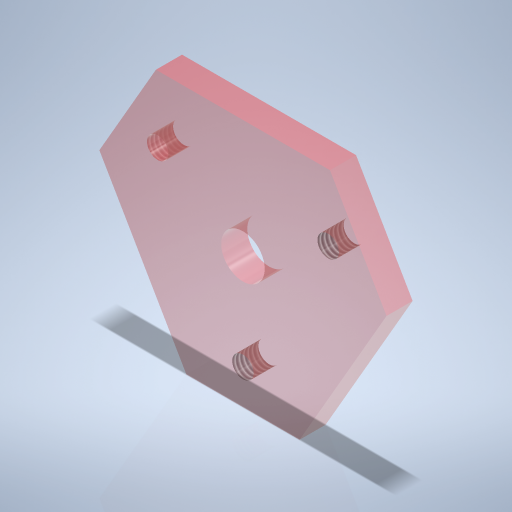
# Autodesk Inventor part: Plate
Saved by Autodesk Inventor 2024 (Build 280153000, 153)
## iProperties
Created: 2024-06-06
Part Number: Plate
Material: Aluminium 6061
Document SubType Name: Modeling
Designer: ffogue
Density: 2.7 g/cm^3
Appearance: Dunkelrot
Author: ffogue
Autodesk Inventor part; units mm, degrees
ref_plane "YZ Plane" through (0, 0, 0) normal (1, 0, 0) x (0, 1, 0)
ref_plane "XZ Plane" through (0, 0, 0) normal (0, 1, 0) x (-1, 0, 0)
ref_plane "XY Plane" through (0, 0, 0) normal (0, 0, 1) x (1, 0, 0)
sketch "Skizze1" plane through (0, 0, 0) normal (0, 1, 0) x (-1, 0, 0)
  line L0 (0, 0) -> (46, 79.6743)
  line L1 (46, 79.6743) -> (-46, 79.6743)
  line L2 (-46, 79.6743) -> (0, 0)
  line L3 (0, 0) -> (0, 79.6743) construction
  line L4 (-46, 79.6743) -> (23, 39.8372) construction
  line L5 (46, 79.6743) -> (-23, 39.8372) construction
  dimension "d0" = 92
  constraints: 12 end point, 3 midpoint, 1 equal length, 1 horizontal, 1 symmetric about line, 1 vertical
  measures "d0" distance of L1.end L0.start
extrude "Extrusion1" add sketch "Skizze1" along normal mid plane 6
sketch "Skizze2" plane through (0, -3, 0) normal (0, -1, 0) x (1, 0, 0)
  line L0 (46, 79.6743) -> (-46, 79.6743) projected
  line L1 (-46, 79.6743) -> (0, 0) projected
  line L2 (0, 0) -> (46, 79.6743) projected
  line L3 (0, 0) -> (0, 0) construction
  line L4 (0, 0) -> (0, 79.6743) construction
  line L5 (-46, 79.6743) -> (0, 0) projected
  line L6 (46, 79.6743) -> (-46, 79.6743) projected
  line L7 (-23, 39.8372) -> (46, 79.6743) construction
  line L8 (23, 39.8372) -> (-46, 79.6743) construction
  line L9 (-33, 57.1577) -> (-20, 79.6743)
  point P0 (-33, 57.1577)
  point P1 (-20, 79.6743)
  point P2 (-26.5, 68.416)
  dimension "d31" = 26
  constraints: 10 end point, 4 midpoint, 3 point on line, 1 perpendicular, 1 vertical
  measures "d31" distance of L9.start L9.end
extrude "Extrusion6" cut sketch "Skizze2" against normal blind 10 contours L9 L1 L0
mirror "Spiegeln1" about plane through (0, 0, 0) normal (1, 0, 0) of "Extrusion6"
sketch "Skizze7" plane through (0, -3, 0) normal (0, -1, 0) x (1, 0, 0)
  line L0 (0, 0) -> (-33, 57.1577) projected
  line L1 (-13, 22.5167) -> (13, 22.5167)
  line L2 (33, 57.1577) -> (0, 0) projected
  dimension "d38" = 26
  constraints: 2 end point, 2 point on line, 1 horizontal
  measures "d38" distance of L1.start L1.end
extrude "Extrusion7" cut sketch "Skizze7" against normal blind 10
sketch "Skizze3" plane through (0, -3, 0) normal (0, -1, 0) x (1, 0, 0)
  line L0 (46, 79.6743) -> (-46, 79.6743) projected
  line L1 (-13, 22.5167) -> (13, 22.5167) projected
  line L2 (-20, 79.6743) -> (-33, 57.1577) projected
  line L3 (33, 57.1577) -> (20, 79.6743) projected
  point P0 (0, 0)
  point P1 (-19.5959, 64.3743)
  point P2 (19.5959, 64.3743)
  point P3 (0, 30.5167)
  point P4 (33.8756, 72.6743)
  point P5 (-26.5, 68.416)
  dimension "d41" = 8
  dimension "d42" = 8
  dimension "d43" = 8
  dimension "d44" = 15.3
  constraints: 1 horizontal alignment, 1 midpoint, 1 vertical alignment
  measures "d41" distance from line of L1 point (0, 30.517)
  measures "d42" distance from line of L2 point (-19.596, 64.374)
  measures "d43" distance from line of L3 point (19.596, 64.374)
  measures "d44" distance from line of point (-19.596, 64.374) L0
hole "Bohrung1" at (-19.5959, -3, 64.3743) at (19.5959, -3, 64.3743) at (0, -3, 30.5167) direction (0, 1, 0) diameter 4.917 depth 6 thread size "M6x1" class "6H" standard "ISO Metric profile"
sketch "Skizze8" plane through (0, -3, 0) normal (0, -1, 0) x (1, 0, 0)
  circle A0 centre (0, 52.5167) radius 5
  line L0 (-13, 22.5167) -> (13, 22.5167) projected
  point P0 (0, 0)
  point P1 (0, 22.5167)
  dimension "d45" = 30
  dimension "d46" = 10
  constraints: 1 centre point, 1 midpoint, 1 vertical alignment
  measures "d45" distance from line of L0 A0.centre
  measures "d46" diameter of A0
extrude "Extrusion8" cut sketch "Skizze8" against normal blind 10
equation "\"d42\" = d41"
equation "\"d43\" = d42"
equation "\"d9\" = d8"
equation "\"d8\" = 8"
